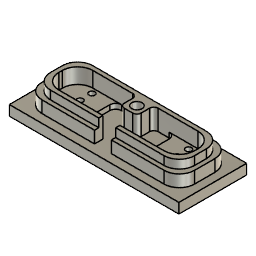
CAM-Model (Autodesk Fusion 360 design; units mm, degrees)
part number: 2025-09-15-18-47-47-813
Autodesk Fusion 360 part; units mm, degrees
sketch "Sketch1" plane through (0, 0, 0) normal (0, 0, 1) x (1, 0, 0)
  line L0 (99.503, -40) -> (-100.497, -40)
  line L1 (-100.497, -40) -> (-100.497, 40)
  line L2 (-100.497, 40) -> (99.503, 40)
  line L3 (99.503, 40) -> (99.503, -40)
  line L4 (99.503, -40) -> (-100.497, 40) construction
  line L5 (-100.497, -40) -> (99.503, 40) construction
  point P0 (-0.497, 0)
  dimension "d1" = 200
  dimension "d2" = 80
  constraint horizontal L0
  constraint perpendicular L0 L1
  constraint parallel L0 L2
  constraint parallel L1 L3
  constraint coincident L4 P0
  constraint coincident L5 P0
  measures "d1" distance of L1.end L2.end
  measures "d2" distance of L0.end L1.end
extrude "Extrude1" add sketch "Sketch1" along normal blind 12
sketch "Sketch2" plane through (0, 0, 12) normal (0, 0, 1) x (-1, 0, 0)
  line L0 (-99.503, -40) -> (100.497, -40)
  line L1 (100.497, -40) -> (100.497, 40)
  line L2 (100.497, 40) -> (-99.503, 40)
  line L3 (-99.503, 40) -> (-99.503, -40)
  line L4 (90, -30) -> (-90, -30)
  line L5 (-90, -30) -> (-90, 30)
  line L6 (-90, 30) -> (-10, 30)
  line L7 (-10, 30) -> (-10, 20)
  line L8 (-10, 20) -> (-80, 20)
  line L9 (-80, 20) -> (-80, -20)
  line L10 (-80, -20) -> (80, -20)
  line L11 (80, -20) -> (80, 20)
  line L12 (80, 20) -> (10, 20)
  line L13 (10, 30) -> (10, 20)
  line L14 (10, 30) -> (90, 30)
  line L15 (90, 30) -> (90, -30)
  line L16 (10, 25) -> (85, 25)
  line L17 (85, 25) -> (85, -25)
  line L18 (85, -25) -> (10, -25)
  line L19 (10, -25) -> (10, 0)
  line L20 (10, 0) -> (-10, 0)
  line L21 (-10, 0) -> (-10, -25)
  line L22 (-10, -25) -> (-85, -25)
  line L23 (-85, -25) -> (-85, 25)
  line L24 (-85, 25) -> (-10, 25)
  line L25 (10, -25) -> (-10, -25)
  constraint perpendicular L1 L4
  constraint perpendicular L4 L5
  constraint perpendicular L5 L6
  constraint perpendicular L6 L7
  constraint perpendicular L7 L8
  constraint perpendicular L6 L9
  constraint perpendicular L7 L10
  constraint perpendicular L10 L11
  constraint perpendicular L11 L12
  constraint perpendicular L12 L13
  constraint perpendicular L13 L14
  constraint perpendicular L4 L15
  constraint midpoint L13 L16.start
  constraint perpendicular L11 L16
  constraint perpendicular L4 L17
  constraint perpendicular L17 L18
  constraint perpendicular L18 L19
  constraint perpendicular L19 L20
  constraint perpendicular L10 L21
  constraint perpendicular L21 L22
  constraint perpendicular L22 L23
  constraint midpoint L7 L24.end
  constraint perpendicular L7 L24
  constraint perpendicular L21 L25
extrude "Extrude2" add sketch "Sketch2" along normal blind 15 contours L10 L11 L12 L13 L16 L17 L18 L19 | L7 L8 L9 L10 L21 L22 L23 L24 | L10 L19 L21 L25 | L10 L19 L20 L21
sketch "Sketch3" plane through (0, 0, 12) normal (0, 0, 1) x (-1, 0, 0)
  line L0 (10, 25) -> (85, 25)
  line L1 (85, 25) -> (85, -25)
  line L2 (85, -25) -> (-85, -25)
  line L3 (-85, -25) -> (-85, 25)
  line L4 (-85, 25) -> (-10, 25)
  line L5 (-10, 25) -> (-10, 20)
  line L6 (-10, 20) -> (-80, 20)
  line L7 (-80, 20) -> (-80, -20)
  line L8 (-80, -20) -> (-10, -20)
  line L9 (-10, -20) -> (-10, 0)
  line L10 (-10, 0) -> (10, 0)
  line L11 (10, 0) -> (10, -20)
  line L12 (10, -20) -> (80, -20)
  line L13 (80, -20) -> (80, 20)
  line L14 (80, 20) -> (10, 20)
  line L15 (10, 20) -> (10, 25)
  line L16 (-99.503, -40) -> (100.497, -40)
  line L17 (100.497, -40) -> (100.497, 40)
  line L18 (100.497, 40) -> (-99.503, 40)
  line L19 (-99.503, 40) -> (-99.503, -40)
  line L20 (90, -30) -> (-90, -30)
  line L21 (-90, -30) -> (-90, 30)
  line L22 (-90, 30) -> (-10, 30)
  line L23 (-10, 30) -> (-10, 25)
  line L24 (10, 25) -> (10, 30)
  line L25 (10, 30) -> (90, 30)
  line L26 (90, 30) -> (90, -30)
  constraint perpendicular L3 L20
  constraint perpendicular L20 L21
  constraint perpendicular L21 L22
  constraint coincident L4.end L5.start
  constraint perpendicular L4 L23
  constraint coincident L0.start L15.end
  constraint perpendicular L0 L24
  constraint perpendicular L24 L25
  constraint perpendicular L20 L26
extrude "Extrude3" add sketch "Sketch3" along normal blind 14 contours L0 L1 L2 L3 L4 L20 L21 L22 L23 L24 L25 L26
extrude "Extrude4" add 1 faces at (3.3333, 6.6667, 27) along direction (0, 0, 1) blind 9
fillet "Fillet1" radius 5 2 edges at (-10, 0, 24) (10, 0, 24)
fillet "Fillet2" radius 5 2 edges at (10, 20, 24) (-10, 20, 24)
fillet "Fillet3" radius 18 12 edges at (-85, -25, 31) (-90, -30, 19) (85, -25, 31) (90, -30, 19) (90, 30, 19) (85, 25, 31) (-90, 30, 19) (-85, 25, 31) (-80, 20, 24) (80, 20, 24) (-80, -20, 24) (80, -20, 24)
sketch "Sketch4" plane through (0, 0, 36) normal (0, 0, 1) x (-1, 0, 0)
  arc A0 (67, -25) -> (85, -7) centre (67, -7) ccw
  line L0 (85, -7) -> (85, 7)
  arc A1 (85, 7) -> (67, 25) centre (67, 7) ccw
  line L1 (67, 25) -> (10, 25)
  line L2 (10, 25) -> (10, 20)
  line L3 (10, 20) -> (62, 20)
  arc A2 (80, 2) -> (62, 20) centre (62, 2) ccw
  line L4 (80, 2) -> (80, -2)
  arc A3 (62, -20) -> (80, -2) centre (62, -2) ccw
  line L5 (62, -20) -> (15, -20)
  arc A4 (10, -15) -> (15, -20) centre (15, -15) ccw
  line L6 (10, -15) -> (10, -5)
  arc A5 (10, -5) -> (5, 0) centre (5, -5) ccw
  line L7 (5, 0) -> (-5, 0)
  arc A6 (-5, 0) -> (-10, -5) centre (-5, -5) ccw
  line L8 (-10, -5) -> (-10, -15)
  arc A7 (-15, -20) -> (-10, -15) centre (-15, -15) ccw
  line L9 (-15, -20) -> (-62, -20)
  arc A8 (-80, -2) -> (-62, -20) centre (-62, -2) ccw
  line L10 (-80, -2) -> (-80, 2)
  arc A9 (-62, 20) -> (-80, 2) centre (-62, 2) ccw
  line L11 (-62, 20) -> (-10, 20)
  line L12 (-10, 20) -> (-10, 25)
  line L13 (-10, 25) -> (-67, 25)
  arc A10 (-67, 25) -> (-85, 7) centre (-67, 7) ccw
  line L14 (-85, 7) -> (-85, -7)
  arc A11 (-85, -7) -> (-67, -25) centre (-67, -7) ccw
  line L15 (-67, -25) -> (67, -25)
  circle A12 centre (0, -10) radius 6.1104
extrude "Extrude5" cut sketch "Sketch4" against normal blind 30 contours A12
sketch "Sketch5" plane through (0, 0, 12) normal (0, 0, 1) x (-1, 0, 0)
  arc A0 (-62, 20) -> (-80, 2) centre (-62, 2) ccw
  line L0 (-80, 2) -> (-80, -2)
  arc A1 (-80, -2) -> (-62, -20) centre (-62, -2) ccw
  line L1 (-62, -20) -> (-15, -20)
  arc A2 (-15, -20) -> (-10, -15) centre (-15, -15) ccw
  line L2 (-10, -15) -> (-10, -5)
  arc A3 (-5, 0) -> (-10, -5) centre (-5, -5) ccw
  line L3 (-5, 0) -> (5, 0)
  arc A4 (10, -5) -> (5, 0) centre (5, -5) ccw
  line L4 (10, -5) -> (10, -15)
  arc A5 (10, -15) -> (15, -20) centre (15, -15) ccw
  line L5 (15, -20) -> (62, -20)
  arc A6 (62, -20) -> (80, -2) centre (62, -2) ccw
  line L6 (80, -2) -> (80, 2)
  arc A7 (80, 2) -> (62, 20) centre (62, 2) ccw
  line L7 (62, 20) -> (10, 20)
  line L8 (10, 20) -> (10, 30)
  line L9 (10, 30) -> (72, 30)
  arc A8 (90, 12) -> (72, 30) centre (72, 12) ccw
  line L10 (90, 12) -> (90, -12)
  arc A9 (72, -30) -> (90, -12) centre (72, -12) ccw
  line L11 (72, -30) -> (-72, -30)
  arc A10 (-90, -12) -> (-72, -30) centre (-72, -12) ccw
  line L12 (-90, -12) -> (-90, 12)
  arc A11 (-72, 30) -> (-90, 12) centre (-72, 12) ccw
  line L13 (-72, 30) -> (-10, 30)
  line L14 (-10, 30) -> (-10, 20)
  line L15 (-10, 20) -> (-62, 20)
  line L16 (-99.503, -40) -> (100.497, -40)
  line L17 (100.497, -40) -> (100.497, 40)
  line L18 (100.497, 40) -> (-99.503, 40)
  line L19 (-99.503, 40) -> (-99.503, -40)
  line L20 (35, 20) -> (35, -20)
  line L21 (-35, 20) -> (-35, -20)
  constraint coincident L7 L20.start
  constraint coincident L5 L20.end
  constraint perpendicular L5 L20
  constraint coincident L15 L21.start
  constraint coincident L1 L21.end
  constraint perpendicular L1 L21
extrude "Extrude6" add sketch "Sketch5" along normal blind 6 contours A0 L0 A1 L1 L15 L21 | L5 A6 L6 A7 L7 L20
fillet "Fillet4" radius 7 4 edges at (-35, 20, 15) (35, 20, 15) (35, -20, 15) (-35, -20, 15)
sketch "Sketch6" plane through (0, 0, 18) normal (0, 0, 1) x (-1, 0, 0)
  line L0 (35, 13) -> (35, -13)
  arc A0 (28, -20) -> (35, -13) centre (28, -13) ccw
  line L1 (28, -20) -> (62, -20)
  arc A1 (62, -20) -> (80, -2) centre (62, -2) ccw
  line L2 (80, -2) -> (80, 2)
  arc A2 (80, 2) -> (62, 20) centre (62, 2) ccw
  line L3 (62, 20) -> (28, 20)
  arc A3 (35, 13) -> (28, 20) centre (28, 13) ccw
  circle A4 centre (57, 0) radius 3.5
  circle A5 centre (57, 13) radius 3.5
  circle A6 centre (57, -14) radius 3.5
  dimension "d23" = 7
  dimension "d24" = 7
  dimension "d25" = 7
  measures "d23" diameter of A4
  measures "d24" diameter of A5
  measures "d25" diameter of A6
sketch "Sketch7" plane through (0, 0, 18) normal (0, 0, 1) x (-1, 0, 0)
  arc A0 (-62, 20) -> (-80, 2) centre (-62, 2) ccw
  line L0 (-80, 2) -> (-80, -2)
  arc A1 (-80, -2) -> (-62, -20) centre (-62, -2) ccw
  line L1 (-62, -20) -> (-28, -20)
  arc A2 (-35, -13) -> (-28, -20) centre (-28, -13) ccw
  line L2 (-35, -13) -> (-35, 13)
  arc A3 (-28, 20) -> (-35, 13) centre (-28, 13) ccw
  line L3 (-28, 20) -> (-62, 20)
  circle A4 centre (-57, 0) radius 3.5
  circle A5 centre (-57, -14) radius 3.5
  circle A6 centre (-57, 13) radius 3.5
  dimension "d26" = 7
  dimension "d27" = 7
  dimension "d28" = 7
  measures "d26" diameter of A4
  measures "d27" diameter of A5
  measures "d28" diameter of A6
extrude "Extrude7" cut sketch "Sketch7" sketch "Sketch6" against normal blind 10 contours A4 | A5 | A6 of sketch 2 contours A4 | A5 | A6
